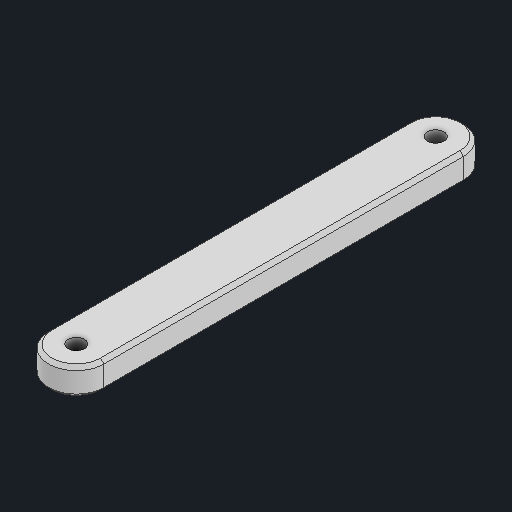
# Autodesk Inventor part: Part2
Saved by Autodesk Inventor 2025.1 (Build 291241020, 241B)
## iProperties
Created: 2025-05-01
Part Number: Part2
Material: Generic
Document SubType Name: Modeling
Designer: Joshua Eah
Density: 1 g/cm^3
Appearance: Default
Author: Joshua Eah
Autodesk Inventor part; units mm, degrees
ref_plane "YZ Plane" through (0, 0, 0) normal (1, 0, 0) x (0, 1, 0)
ref_plane "XZ Plane" through (0, 0, 0) normal (0, 1, 0) x (-1, 0, 0)
ref_plane "XY Plane" through (0, 0, 0) normal (0, 0, 1) x (1, 0, 0)
sketch "Sketch1" plane through (0, 0, 0) normal (0, 1, 0) x (-1, 0, 0)
  line L0 (0, 0) -> (-10.16, 0)
  line L1 (-10.16, 0) -> (-10.16, -76.2)
  line L2 (-10.16, -76.2) -> (0, -76.2)
  line L3 (0, -76.2) -> (0, 0)
  line L4 (-5.08, -76.2) -> (-5.08, 0) construction
  circle A0 centre (-5.08, -71.12) radius 1.5
  circle A1 centre (-5.08, -5.08) radius 1.5
  dimension "d0" = 10.16
  dimension "d1" = 76.2
  dimension "d2" = 3
  dimension "d3" = 3
  dimension "d4" = 5.08
  dimension "d5" = 5.08
  constraints: 10 end point, 2 centre point, 2 midpoint, 2 parallel, 2 point on line, 1 horizontal, 1 perpendicular
  measures "d0" distance of L2.end L1.end
  measures "d1" distance of L1.end L0.end
  measures "d2" diameter of A0
  measures "d3" diameter of A1
  measures "d4" distance from line of L2 A0.centre
  measures "d5" distance from line of L0 A1.centre
extrude "Extrusion1" add sketch "Sketch1" along normal blind 5
fillet "Fillet1" radius 5.08 4 edges at (10.16, 2.5, 0) (0, 2.5, 0) (10.16, 2.5, -76.2) (0, 2.5, -76.2)
chamfer "Chamfer1" distance 0.635 angle 45 12 edges at (10.16, 5, -38.1) (8.6721, 5, -74.7121) (8.6721, 5, -1.4879) (0, 5, -38.1) (1.4879, 5, -1.4879) (1.4879, 5, -74.7121) (10.16, 0, -38.1) (8.6721, 0, -74.7121) (8.6721, 0, -1.4879) (1.4879, 0, -1.4879) (0, 0, -38.1) (1.4879, 0, -74.7121)
equation "\"d4\" = 0.5 * d0"
equation "\"d5\" = d4"
body "Solid1"
